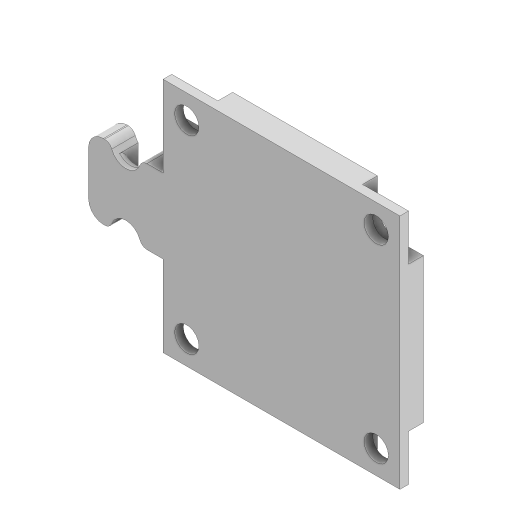
# Autodesk Inventor part: lna605_base
Saved by Autodesk Inventor 2023 (Build 270158000, 158)
## iProperties
Created: 2024-05-13
Part Number: lna605_base
Material: Generic
Document SubType Name: Modeling
Designer: Thomas
Density: 1 g/cm^3
Appearance: Default
Author: Thomas
Autodesk Inventor part; units mm, degrees
ref_plane "YZ Plane" through (0, 0, 0) normal (1, 0, 0) x (0, 1, 0)
ref_plane "XZ Plane" through (0, 0, 0) normal (0, 1, 0) x (-1, 0, 0)
ref_plane "XY Plane" through (0, 0, 0) normal (0, 0, 1) x (1, 0, 0)
sketch "Sketch1" plane through (0, 0, 0) normal (0, 0, 1) x (1, 0, 0)
  line L0 (0, 0) -> (31.75, 0)
  line L1 (31.75, 0) -> (31.75, 31.75)
  line L2 (31.75, 31.75) -> (0, 31.75)
  line L3 (0, 31.75) -> (0, 0)
  line L4 (0, 0) -> (0, 31.75)
  line L5 (0, 20.875) -> (-10, 20.875)
  line L6 (-10, 20.875) -> (-10, 10.875)
  line L7 (-10, 10.875) -> (0, 10.875)
  line L8 (0, 10.875) -> (0, 20.875)
  circle A0 centre (-5, 20.875) radius 2
  circle A1 centre (-5, 10.875) radius 2
  point P0 (-10, 15.875)
  point P1 (0, 15.875)
  point P2 (-7, 10.875)
  point P3 (-3, 10.875)
  point P4 (-3, 20.875)
  point P5 (-7, 20.875)
  dimension "d0" = 31.75
  dimension "d1" = 31.75
  dimension "d19" = 10
  dimension "d20" = 4
  dimension "d21" = 4
  dimension "d22" = 10
  dimension "d23" = 0
  constraints: 18 end point, 4 midpoint, 4 parallel, 2 centre point, 2 horizontal, 2 perpendicular, 1 point on line
  measures "d0" distance of L2.end L1.end
  measures "d1" distance of L1.end L0.end
  measures "d19" distance between parallel lines of L3 L6
  measures "d20" diameter of A0
  measures "d21" diameter of A1
  measures "d22" distance of L5.end L6.end
  measures "d23" vertical distance of point (-10, 15.875) point (0, 15.875)
extrude "Extrusion1" add sketch "Sketch1" against normal blind 3.15 contours L3 L2 L1 L0 | L7 A1 L6 L5 A0 L3
sketch "Sketch2" plane through (0, 0, -3.15) normal (0, 0, -1) x (-1, 0, 0)
  circle A0 centre (-28.575, 28.575) radius 1.632
  circle A1 centre (-28.575, 28.575) radius 3
  line L0 (-28.575, 28.575) -> (-3.175, 28.575) construction
  line L1 (-3.175, 28.575) -> (-3.175, 3.175) construction
  line L2 (-3.175, 3.175) -> (-28.575, 3.175) construction
  line L3 (-28.575, 3.175) -> (-28.575, 28.575) construction
  line L4 (-31.75, 31.75) -> (-31.75, 0) projected
  line L5 (0, 31.75) -> (-31.75, 31.75) projected
  line L6 (-25.575, 28.575) -> (-25.575, 31.75)
  line L7 (-28.575, 25.575) -> (-31.75, 25.575)
  line L8 (-15.875, 28.575) -> (-15.875, 3.175) construction
  line L9 (-3.175, 15.875) -> (-28.575, 15.875) construction
  line L10 (-25.575, 3.175) -> (-25.575, 0)
  circle A2 centre (-28.575, 3.175) radius 1.632
  circle A3 centre (-28.575, 3.175) radius 3
  line L11 (-28.575, 6.175) -> (-31.75, 6.175)
  line L12 (-3.175, 6.175) -> (0, 6.175)
  circle A4 centre (-3.175, 3.175) radius 1.632
  circle A5 centre (-3.175, 3.175) radius 3
  line L13 (-6.175, 3.175) -> (-6.175, 0)
  line L14 (-6.175, 28.575) -> (-6.175, 31.75)
  circle A6 centre (-3.175, 28.575) radius 1.632
  circle A7 centre (-3.175, 28.575) radius 3
  line L15 (-3.175, 25.575) -> (0, 25.575)
  line L16 (-31.75, 0) -> (0, 0) projected
  line L17 (0, 20.875) -> (0, 31.75) projected
  line L18 (0, 0) -> (0, 10.875) projected
  point P0 (-31.75, 15.875)
  point P1 (10, 31.75)
  point P2 (-15.875, 15.875)
  point P3 (-15.875, 15.875)
  point P4 (10, 0)
  dimension "d5" = 3.2639
  dimension "d6" = 6
  dimension "d7" = 25.4
  dimension "d8" = 25.4
  dimension "d9" = 3.175
  dimension "d10" = 3.175
  dimension "d13" = 360
  constraints: 28 end point, 8 centre point, 8 point on circle, 6 midpoint, 5 coincident, 3 perpendicular, 3 point on line, 2 parallel, 1 horizontal, 1 tangent, 41 other
  measures "d5" diameter of A0
  measures "d6" diameter of A1
  measures "d7" distance of L1.end L2.end
  measures "d8" distance of L0.end L1.end
  measures "d9" distance from line of point (-31.75, 15.875) L3
  measures "d10" distance between parallel lines of L0 L5
extrude "Extrusion2" cut sketch "Sketch2" against normal blind 2
extrude "Extrusion3" cut sketch "Sketch2" against normal through all contours A0 | A2 | A4 | A6
sketch "Sketch3" plane through (0, 0, -3.15) normal (0, 0, -1) x (-1, 0, 0)
  line L0 (3.5, 20.875) -> (6.5, 20.875)
  line L1 (6.5, 20.875) -> (6.5, 10.875)
  line L2 (6.5, 10.875) -> (3.5, 10.875)
  line L3 (3.5, 10.875) -> (3.5, 20.875)
  line L4 (7, 10.875) -> (10, 10.875) projected
  point P0 (0, 0)
  point P1 (3, 20.875)
  point P2 (3, 10.875)
  dimension "d26" = 0.5
  dimension "d27" = 0.5
  dimension "d28" = 3
  constraints: 8 end point, 2 parallel, 2 point on line, 1 horizontal, 1 perpendicular
  measures "d26" distance from line of L4.start L1
  measures "d27" distance from line of point (3, 10.875) L3
  measures "d28" distance of L1.end L2.end
extrude "Extrusion4" cut sketch "Sketch3" against normal blind 1.5
fillet "Fillet1" radius 1 6 edges at (-5, 18.875, -1.65) (-3, 20.875, -1.575) (-7, 20.875, -1.575) (-5, 12.875, -1.65) (-7, 10.875, -1.575) (-3, 10.875, -1.575)
fillet "Fillet2" radius 2 2 edges at (-10, 20.875, -1.575) (-10, 10.875, -1.575)
body "Solid1"
